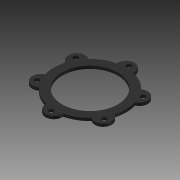
# Autodesk Inventor part: rubber ring
Saved by Autodesk Inventor 2015 (Build 190159000, 159)
## iProperties
Created: 2015-02-28
Part Number: rubber ring
Material: Generic
Document SubType Name: Modeling
Designer: Qiuyang
Density: 1 g/cm^3
Appearance: Default
Author: Qiuyang
Autodesk Inventor part; units mm, degrees
ref_plane "YZ Plane" through (0, 0, 0) normal (1, 0, 0) x (0, 1, 0)
ref_plane "XZ Plane" through (0, 0, 0) normal (0, 1, 0) x (-1, 0, 0)
ref_plane "XY Plane" through (0, 0, 0) normal (0, 0, 1) x (1, 0, 0)
sketch "Sketch11" plane through (0, 0, 0) normal (0, 1, 0) x (-1, 0, 0)
  circle A0 centre (0, 0) radius 31.75
  circle A1 centre (0, 0) radius 41.275
  dimension "d79" = 63.5
  dimension "d80" = 82.55
  constraints: 2 centre point, 2 coincident
  measures "d79" diameter of A0
  measures "d80" diameter of A1
extrude "Extrusion10" add sketch "Sketch11" along normal blind 3.175
sketch "Sketch12" plane through (0, 3.175, 0) normal (0, 1, 0) x (1, 0, 0)
  circle A0 centre (0, 0) radius 41.275 projected
  circle A1 centre (0, -41.275) radius 9.5284
  circle A2 centre (35.7452, -20.6375) radius 9.5284
  circle A3 centre (35.7452, 20.6375) radius 9.5284
  circle A4 centre (0, 41.275) radius 9.5284
  circle A5 centre (-35.7452, 20.6375) radius 9.5284
  circle A6 centre (-35.7452, -20.6375) radius 9.5284
  dimension "d85" = 360
  constraints: 6 centre point, 1 vertical alignment, 14 other
extrude "Extrusion11" add sketch "Sketch12" against normal blind 3.175 contours A3 A0 | A0 A3 | A2 A0 | A0 A2 | A4 A0 | A0 A4 | A1 A0 | A0 A1 | A5 A0 | A0 A5 | A6 A0 | A0 A6
sketch "Sketch13" plane through (0, 3.175, 0) normal (0, 1, 0) x (1, 0, 0)
  circle A0 centre (0, -44.45) radius 2.794
  circle A1 centre (38.4948, -22.225) radius 2.794
  circle A2 centre (38.4948, 22.225) radius 2.794
  circle A3 centre (0, 44.45) radius 2.794
  circle A4 centre (-38.4948, 22.225) radius 2.794
  circle A5 centre (-38.4948, -22.225) radius 2.794
  point P0 (0, 0)
  dimension "d89" = 5.588
  dimension "d92" = 360
  constraints: 6 centre point, 13 other
  measures "d89" diameter of A0
extrude "Extrusion12" cut sketch "Sketch13" against normal blind 3.175
body "Solid3"
